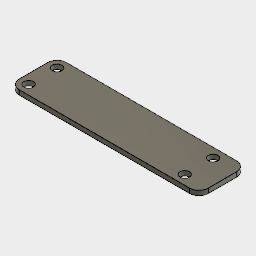
Direct Edit_CSA011010 (Autodesk Fusion 360 design; units mm, degrees)
Autodesk Fusion 360 part; units mm, degrees
sketch "Sketch1" plane through (0, 0, 0) normal (0, 1, 0) x (1, 0, 0)
  line L0 (100, 25) -> (-100, 25)
  line L1 (-100, 25) -> (-100, -25)
  line L2 (-100, -25) -> (100, -25)
  line L3 (100, -25) -> (100, 25)
  line L4 (100, 25) -> (-100, -25) construction
  line L5 (-100, 25) -> (100, -25) construction
  dimension "d1" = 200
  dimension "d2" = 50
  measures "d1" distance of L1.end L2.end
  measures "d2" distance of L0.end L1.end
extrude "Extrude1" add sketch "Sketch1" along normal blind 5
fillet "Fillet1" radius 10 4 edges at (-100, 2.5, 25) (-100, 2.5, -25) (100, 2.5, -25) (100, 2.5, 25)
sketch "Sketch2" plane through (0, 5, 0) normal (0, 1, 0) x (-1, 0, 0)
  arc A0 (-90, 25) -> (-100, 15) centre (-90, 15) ccw
  line L0 (-100, 15) -> (-100, -15)
  arc A1 (-100, -15) -> (-90, -25) centre (-90, -15) ccw
  line L1 (-90, -25) -> (90, -25)
  arc A2 (90, -25) -> (100, -15) centre (90, -15) ccw
  line L2 (100, -15) -> (100, 15)
  arc A3 (100, 15) -> (90, 25) centre (90, 15) ccw
  line L3 (90, 25) -> (-90, 25)
  circle A4 centre (90, -15) radius 5
  circle A5 centre (90, 15) radius 5
  circle A6 centre (-75, -15) radius 5
  circle A7 centre (-75, 15) radius 5
  dimension "d6" = 10
  dimension "d7" = 15
  measures "d6" diameter of A4
  measures "d7" distance of A1.end A6.centre
extrude "Extrude2" cut sketch "Sketch2" against normal through all contours A4 | A5 | A6 | A7
